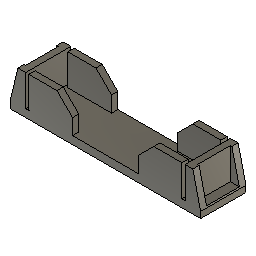
AAA Battery Holder v1 (Autodesk Fusion 360 design; units mm, degrees)
Autodesk Fusion 360 part; units mm, degrees
sketch "Sketch1" plane through (0, 0, 0) normal (0, 0, 1) x (1, 0, 0)
  line L0 (0, 0) -> (61, 0)
  line L1 (61, 0) -> (61, 14.5)
  line L2 (61, 14.5) -> (0, 14.5)
  line L3 (0, 14.5) -> (0, 0)
  dimension "d1" = 61
  dimension "d2" = 14.5
  constraint horizontal L0
  constraint vertical L1
  constraint horizontal L2
  constraint vertical L3
  constraint coincident L0.start L3.end
  measures "d1" distance of L0.start L0.end
  measures "d2" distance of L0.start L2.end
extrude "Extrude1" add sketch "Sketch1" along normal blind 2.5
sketch "Sketch2" plane through (0, 0, 2.5) normal (0, 0, 1) x (-1, 0, 0)
  line L0 (0, -14.5) -> (0, 0)
  line L1 (0, 0) -> (-61, 0)
  line L2 (-61, 0) -> (-61, -14.5)
  line L3 (-61, -14.5) -> (0, -14.5)
  line L4 (-5, -24.7983) -> (-5, 20) construction
  line L5 (-56, -25) -> (-56, 25) construction
  line L6 (12, -12.5) -> (-78, -12.5) construction
  line L7 (12, -2) -> (-79, -2) construction
  line L8 (-5, -14.5) -> (-3, -14.5)
  line L9 (-3, -14.5) -> (-3, 0)
  line L10 (-3, 0) -> (-5, 0)
  line L11 (-5, 0) -> (-5, -14.5)
  line L12 (-56, -14.5) -> (-58, -14.5)
  line L13 (-58, -14.5) -> (-58, 0)
  line L14 (-58, 0) -> (-56, 0)
  line L15 (-56, 0) -> (-56, -14.5)
  line L16 (-6, -14.5) -> (-20, -14.5)
  line L17 (-20, -14.5) -> (-20, -12.5)
  line L18 (-20, -12.5) -> (-6, -12.5)
  line L19 (-6, -12.5) -> (-6, -14.5)
  line L20 (-6, -2) -> (-20, -2)
  line L21 (-20, -2) -> (-20, 0)
  line L22 (-20, 0) -> (-6, 0)
  line L23 (-6, 0) -> (-6, -2)
  line L24 (-55, -14.5) -> (-41, -14.5)
  line L25 (-41, -14.5) -> (-41, -12.5)
  line L26 (-41, -12.5) -> (-55, -12.5)
  line L27 (-55, -12.5) -> (-55, -14.5)
  line L28 (-41, -2) -> (-55, -2)
  line L29 (-55, -2) -> (-55, 0)
  line L30 (-55, 0) -> (-41, 0)
  line L31 (-41, 0) -> (-41, -2)
  line L32 (-3, -14.5) -> (0, -14.5)
  line L33 (0, -14.5) -> (0, -12.5)
  line L34 (0, -12.5) -> (-3, -12.5)
  line L35 (-3, -12.5) -> (-3, -14.5)
  line L36 (-58, -14.5) -> (-61, -14.5)
  line L37 (-61, -14.5) -> (-61, -12.5)
  line L38 (-61, -12.5) -> (-58, -12.5)
  line L39 (-58, -12.5) -> (-58, -14.5)
  line L40 (-58, -2) -> (-61, -2)
  line L41 (-61, -2) -> (-61, 0)
  line L42 (-61, 0) -> (-58, 0)
  line L43 (-58, 0) -> (-58, -2)
  line L44 (-3, -2) -> (0, -2)
  line L45 (0, -2) -> (0, 0)
  line L46 (0, 0) -> (-3, 0)
  line L47 (-3, 0) -> (-3, -2)
  dimension "d5" = 51
  dimension "d6" = 5
  dimension "d7" = 10.5
  dimension "d8" = 2
  dimension "d9" = 14
  dimension "d10" = 14
  dimension "d11" = 14
  dimension "d12" = 14
  dimension "d13" = 1
  dimension "d14" = 1
  dimension "d15" = 1
  dimension "d16" = 1
  constraint perpendicular L3 L4
  constraint vertical L5
  constraint perpendicular L2 L6
  constraint perpendicular L2 L7
  constraint horizontal L8
  constraint vertical L9
  constraint horizontal L10
  constraint vertical L11
  constraint coincident L1 L9.end
  constraint coincident L3 L8.start
  constraint coincident L4 L8.start
  constraint horizontal L12
  constraint vertical L13
  constraint horizontal L14
  constraint vertical L15
  constraint coincident L5 L12.start
  constraint coincident L3 L12.start
  constraint horizontal L16
  constraint vertical L17
  constraint horizontal L18
  constraint vertical L19
  constraint coincident L3 L16.start
  constraint horizontal L20
  constraint vertical L21
  constraint horizontal L22
  constraint vertical L23
  constraint coincident L7 L20.start
  constraint horizontal L24
  constraint vertical L25
  constraint horizontal L26
  constraint vertical L27
  constraint coincident L3 L24.start
  constraint horizontal L28
  constraint vertical L29
  constraint horizontal L30
  constraint vertical L31
  constraint coincident L7 L28.start
  constraint horizontal L32
  constraint vertical L33
  constraint horizontal L34
  constraint vertical L35
  constraint coincident L0 L33.end
  constraint coincident L6 L33.end
  constraint horizontal L36
  constraint vertical L37
  constraint horizontal L38
  constraint vertical L39
  constraint coincident L6 L37.end
  constraint coincident L2 L37.end
  constraint horizontal L40
  constraint vertical L41
  constraint horizontal L42
  constraint vertical L43
  constraint coincident L1.end L2.start
  constraint coincident L13 L40.start
  constraint coincident L7 L40.start
  constraint horizontal L44
  constraint vertical L45
  constraint horizontal L46
  constraint vertical L47
  constraint coincident L0.end L1.start
  constraint coincident L7 L44.start
  constraint coincident L9 L44.start
  measures "d5" distance of L4 L5
  measures "d6" distance of L0 L4
  measures "d7" distance of L6 L7
  measures "d8" distance of L3 L6
  measures "d9" distance of L16.start L16.end
  measures "d10" distance of L20.start L20.end
  measures "d11" distance of L24.start L24.end
  measures "d12" distance of L28.start L28.end
  measures "d13" distance of L11 L19
  measures "d14" distance of L4 L23
  measures "d15" distance of L15 L27
  measures "d16" distance of L15 L29
extrude "Extrude2" add sketch "Sketch2" along normal blind 10 contours L0 L3 L9 L32 L33 L34 L35 | L1 L3 L8 L9 L10 L11 L35 L47 | L0 L1 L9 L44 L45 L46 L47 | L3 L16 L17 L18 L19 | L1 L20 L21 L22 L23 | L3 L24 L25 L26 L27 | L1 L28 L29 L30 L31 | L1 L3 L12 L13 L14 L15 L39 L43 | L2 L3 L13 L36 L37 L38 L39 | L1 L2 L13 L40 L41 L42 L43
sketch "Sketch3" plane through (0, 0, 0) normal (0, -1, 0) x (1, 0, 0)
  line L0 (0, 0) -> (61, 0)
  line L1 (61, 0) -> (61, 12.5)
  line L2 (61, 12.5) -> (56, 12.5)
  line L3 (56, 12.5) -> (56, 2.5)
  line L4 (56, 2.5) -> (55, 2.5)
  line L5 (55, 2.5) -> (55, 12.5)
  line L6 (55, 12.5) -> (41, 12.5)
  line L7 (41, 12.5) -> (41, 2.5)
  line L8 (41, 2.5) -> (20, 2.5)
  line L9 (20, 2.5) -> (20, 12.5)
  line L10 (20, 12.5) -> (6, 12.5)
  line L11 (6, 12.5) -> (6, 2.5)
  line L12 (6, 2.5) -> (5, 2.5)
  line L13 (5, 2.5) -> (5, 12.5)
  line L14 (5, 12.5) -> (0, 12.5)
  line L15 (0, 12.5) -> (0, 0)
  line L16 (2.5, 12.5) -> (0, 2)
  line L17 (0, 12.5) -> (0, 2)
  line L18 (0, 12.5) -> (2.5, 12.5)
  line L19 (58.5, 12.5) -> (61, 2)
  line L20 (61, 2) -> (61, 12.5)
  line L21 (61, 12.5) -> (58.5, 12.5)
  constraint midpoint L14 L16.start
  constraint coincident L15 L16.end
  constraint coincident L14.end L15.start
  constraint perpendicular L14 L17
  constraint midpoint L2 L19.start
  constraint coincident L1 L19.end
  constraint coincident L1.end L2.start
extrude "Extrude3" cut sketch "Sketch3" against normal blind 68 contours L14 L15 L16 L17 L18 | L1 L2 L19 L20 L21
chamfer "Chamfer1" distance 5 angle 45 4 edges at (20, 13.5, 12.5) (41, 13.5, 12.5) (41, 1, 12.5) (20, 1, 12.5)
